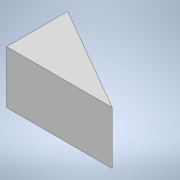
# Autodesk Inventor part: 30-degreeAngleForChopSaw
Saved by Autodesk Inventor 2020.2 (Build 242310000, 310)
## iProperties
Created: 2020-01-19
Part Number: 30-degreeAngleForChopSaw
Material: Generic
Document SubType Name: Modeling
Designer: robst
Density: 1 g/cm^3
Appearance: Default
Author: robst
Autodesk Inventor part; units mm, degrees
ref_plane "YZ Plane" through (0, 0, 0) normal (1, 0, 0) x (0, 1, 0)
ref_plane "XZ Plane" through (0, 0, 0) normal (0, 1, 0) x (-1, 0, 0)
ref_plane "XY Plane" through (0, 0, 0) normal (0, 0, 1) x (1, 0, 0)
sketch "Sketch1" plane through (0, 0, 0) normal (0, 1, 0) x (-1, 0, 0)
  line L0 (0, 0) -> (101.6, 0)
  line L1 (0, 0) -> (101.6, -58.6588)
  line L2 (101.6, 0) -> (101.6, -58.6588)
  dimension "d0" = 101.6
  dimension "d1" = 30
  constraints: 6 end point, 1 horizontal, 1 vertical
  measures "d0" distance of L0.start L0.end
  measures "d1" angle of L0 L1
extrude "Extrusion1" add sketch "Sketch1" along normal blind 50.8
body "Solid1"
